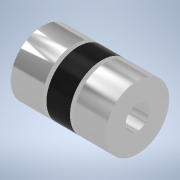
# Autodesk Inventor part: Coupling_SOH_16C_6_6
Saved by Autodesk Inventor 2021 (Build 250183000, 183)
## iProperties
Created: 2020-11-17
Part Number: Coupling_SOH_16C_6_6
Material: アルミニウム 6061
Document SubType Name: Modeling
Designer: yuta2
Density: 2.7 g/cm^3
Appearance: アルミニウム - フラット
Author: yuta2
Autodesk Inventor part; units mm, degrees
ref_plane "YZ Plane" through (0, 0, 0) normal (1, 0, 0) x (0, 1, 0)
ref_plane "XZ Plane" through (0, 0, 0) normal (0, 1, 0) x (-1, 0, 0)
ref_plane "XY Plane" through (0, 0, 0) normal (0, 0, 1) x (1, 0, 0)
sketch "スケッチ1" plane through (0, 0, 0) normal (0, 0, 1) x (1, 0, 0)
  line L0 (0, 0) -> (23.9, 0)
  line L1 (23.9, 0) -> (23.9, 8)
  line L2 (23.9, 8) -> (0, 8)
  line L3 (0, 8) -> (0, 0)
  line L4 (0, 0) -> (11, 0)
  line L5 (11, 0) -> (11, 3)
  line L6 (11, 3) -> (0, 3)
  line L7 (0, 3) -> (0, 0)
  line L8 (23.9, 0) -> (12.9, 0)
  line L9 (12.9, 0) -> (12.9, 3)
  line L10 (12.9, 3) -> (23.9, 3)
  line L11 (23.9, 3) -> (23.9, 0)
  line L12 (9, 8) -> (14.9, 8)
  line L13 (14.9, 8) -> (14.9, 0)
  line L14 (14.9, 0) -> (9, 0)
  line L15 (9, 0) -> (9, 8)
  line L16 (9, 8) -> (8, 8)
  line L17 (8, 8) -> (8, 4)
  line L18 (8, 4) -> (9, 4)
  line L19 (9, 4) -> (9, 8)
  line L20 (14.9, 8) -> (15.9, 8)
  line L21 (15.9, 8) -> (15.9, 4)
  line L22 (15.9, 4) -> (14.9, 4)
  line L23 (14.9, 4) -> (14.9, 8)
  dimension "d0" = 8
  dimension "d1" = 23.9
  dimension "d2" = 11
  dimension "d3" = 3
  dimension "d4" = 11
  dimension "d5" = 3
  dimension "d6" = 2
  dimension "d7" = 2
  dimension "d8" = 1
  dimension "d9" = 4
  dimension "d10" = 1
  dimension "d11" = 4
  constraints: 48 end point, 12 parallel, 6 horizontal, 6 perpendicular, 2 point on line
  measures "d0" distance of L0.end L1.end
  measures "d1" distance of L1.end L2.end
  measures "d2" distance of L6.end L5.end
  measures "d3" distance of L5.end L4.end
  measures "d4" distance of L9.end L10.end
  measures "d5" distance of L8.end L9.end
  measures "d6" distance between parallel lines of L15 L5
  measures "d7" distance between parallel lines of L13 L9
  measures "d8" distance of L18.end L17.end
  measures "d9" distance of L17.end L16.end
  measures "d10" distance of L21.end L22.end
  measures "d11" distance of L20.end L21.end
revolve "回転1" add sketch "スケッチ1" angle 360 about axis through (0, 0, 0) along (1, 0, 0) contours L3 L2 L17 L18 L15 L6 | L5 L6 L15 L2 L13 L10 L9 L0 | L13 L22 L21 L2 L1 L10
